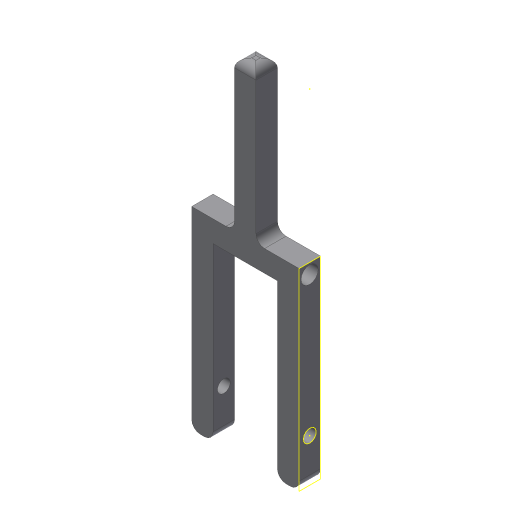
# Autodesk Inventor part: Hebel
Saved by Autodesk Inventor 2023 (Build 270158000, 158)
## iProperties
Created: 2025-01-21
Part Number: Hebel
Material: Generisch
Document SubType Name: Modeling
Designer: abdel
Density: 1 g/cm^3
Appearance: Vorgabe
Author: abdel
Autodesk Inventor part; units mm, degrees
ref_plane "YZ Plane" through (0, 0, 0) normal (1, 0, 0) x (0, 1, 0)
ref_plane "XZ Plane" through (0, 0, 0) normal (0, 1, 0) x (-1, 0, 0)
ref_plane "XY Plane" through (0, 0, 0) normal (0, 0, 1) x (1, 0, 0)
sketch "Skizze1" plane through (0, 0, 0) normal (0, 0, 1) x (1, 0, 0)
  line L0 (-2.5, -2.5) -> (2.5, -2.5)
  line L1 (2.5, -2.5) -> (2.5, 2.5)
  line L2 (2.5, 2.5) -> (-2.5, 2.5)
  line L3 (-2.5, 2.5) -> (-2.5, -2.5)
  line L4 (-2.5, -2.5) -> (2.5, 2.5) construction
  line L5 (2.5, -2.5) -> (-2.5, 2.5) construction
  point P0 (0, 0)
  dimension "d0" = 5
  dimension "d1" = 5
  constraints: 12 end point, 2 midpoint, 2 parallel, 1 horizontal, 1 perpendicular
  measures "d0" distance of L2.end L1.end
  measures "d1" distance of L1.end L0.end
extrude "Extrusion1" add sketch "Skizze1" against normal blind 40
sketch "Skizze3" plane through (-2.5, -2.5, 0) normal (-1, 0, 0) x (0, 0, 1)
  line L0 (0, 5) -> (-40, 5) projected
  line L1 (-40, 0) -> (-40, 5) projected
  line L2 (0, 0) -> (-40, 0) projected
  line L3 (-35, 5) -> (-40, 5)
  line L4 (-40, 5) -> (-40, 0)
  line L5 (-40, 0) -> (-35, 0)
  line L6 (-35, 0) -> (-35, 5)
  line L7 (-35, 5) -> (-40, 0) construction
  line L8 (-40, 5) -> (-35, 0) construction
  point P0 (0, 2.5)
  point P1 (-37.5, 2.5)
  point P2 (-40, 2.5)
  point P3 (-35, 0)
  point P4 (-35, 5)
  dimension "d14" = 5
  dimension "d15" = 5
  constraints: 12 end point, 4 midpoint, 2 parallel, 1 horizontal, 1 perpendicular
  measures "d14" distance of L5.end L4.end
  measures "d15" distance of L4.end L3.end
sketch "Skizze4" plane through (2.5, -2.5, 0) normal (1, 0, 0) x (0, 0, -1)
  line L0 (0, 0) -> (40, 0) projected
  line L1 (40, 5) -> (40, 0) projected
  line L2 (0, 5) -> (40, 5) projected
  line L3 (35, 5) -> (40, 5)
  line L4 (40, 5) -> (40, 0)
  line L5 (40, 0) -> (35, 0)
  line L6 (35, 0) -> (35, 5)
  line L7 (35, 5) -> (40, 0) construction
  line L8 (40, 5) -> (35, 0) construction
  point P0 (0, 2.5)
  point P1 (37.5, 2.5)
  point P2 (40, 2.5)
  point P3 (35, 5)
  point P4 (35, 0)
  dimension "d16" = 5
  dimension "d17" = 5
  constraints: 12 end point, 4 midpoint, 2 parallel, 1 horizontal, 1 perpendicular
  measures "d16" distance of L4.end L5.end
  measures "d17" distance of L3.end L4.end
extrude "Extrusion2" add sketch "Skizze4" along normal blind 10
extrude "Extrusion3" add sketch "Skizze3" along normal blind 10
sketch "Skizze5" plane through (0, 0, -40) normal (0, 0, -1) x (-1, 0, 0)
  line L0 (12.5, -2.5) -> (-12.5, -2.5) projected
  line L1 (12.5, 2.5) -> (12.5, -2.5) projected
  line L2 (-12.5, 2.5) -> (12.5, 2.5) projected
  line L3 (-12.5, -2.5) -> (-12.5, 2.5) projected
  line L4 (12.5, -2.5) -> (7.5, -2.5)
  line L5 (7.5, -2.5) -> (7.5, 2.5)
  line L6 (7.5, 2.5) -> (12.5, 2.5)
  line L7 (12.5, 2.5) -> (12.5, -2.5)
  line L8 (12.5, -2.5) -> (7.5, 2.5) construction
  line L9 (7.5, -2.5) -> (12.5, 2.5) construction
  line L10 (-7.5, 2.5) -> (-12.5, 2.5)
  line L11 (-12.5, 2.5) -> (-12.5, -2.5)
  line L12 (-12.5, -2.5) -> (-7.5, -2.5)
  line L13 (-7.5, -2.5) -> (-7.5, 2.5)
  line L14 (-7.5, 2.5) -> (-12.5, -2.5) construction
  line L15 (-12.5, 2.5) -> (-7.5, -2.5) construction
  point P0 (0, 0)
  point P1 (10, 0)
  point P2 (-10, 0)
  point P3 (12.5, 0)
  point P4 (-12.5, 0)
  point P5 (7.5, 2.5)
  dimension "d22" = 5
  dimension "d23" = 5
  dimension "d24" = 5
  dimension "d25" = 5
  constraints: 24 end point, 8 midpoint, 4 parallel, 2 horizontal, 2 perpendicular
  measures "d22" distance of L5.end L6.end
  measures "d23" distance of L4.end L5.end
  measures "d24" distance of L12.end L11.end
  measures "d25" distance of L11.end L10.end
extrude "Extrusion4" add sketch "Skizze5" along normal blind 40 contours L0 L5 L2 L1 | L0 L3 L2 L13
sketch "Skizze6" plane through (-12.5, -2.5, 0) normal (-1, 0, 0) x (0, 0, 1)
  line L0 (-80, 0) -> (-80, 5) projected
  line L1 (-35, 0) -> (-80, 0) projected
  point P0 (0, 2.5)
  point P1 (-70, 2.5)
  point P2 (-80, 2.5)
  dimension "d35" = 10
  dimension "d36" = 2.5
  constraints: 1 midpoint
  measures "d35" distance of point (-80, 2.5) point (-70, 2.5)
  measures "d36" distance from line of L1 point (-70, 2.5)
hole "Bohrung2" at (-12.5, 0, -70) direction (1, 0, 0) diameter 3 end through all
sketch "Skizze7" plane through (12.5, -2.5, 0) normal (1, 0, 0) x (0, 0, -1)
  circle A0 centre (70, 2.5) radius 1.5 projected
  line L0 (35, 0) -> (80, 0) projected
  line L1 (80, 5) -> (80, 0) projected
  line L2 (35, 5) -> (80, 5) projected
  line L3 (35, 5) -> (35, 0) projected
  point P0 (0, 2.5)
sketch "Skizze8" plane through (-12.5, -2.5, 0) normal (-1, 0, 0) x (0, 0, 1)
  line L0 (-35, 0) -> (-80, 0) projected
  line L1 (-35, 0) -> (-35, 5) projected
  point P0 (0, 2.5)
  point P1 (-37.5, 2.5)
  dimension "d44" = 2.5
  dimension "d45" = 2.5
  measures "d44" distance from line of point (-37.5, 2.5) L1
  measures "d45" distance from line of L0 point (-37.5, 2.5)
hole "Bohrung1" at (-12.5, 0, -37.5) direction (1, 0, 0) diameter 4 end through all
fillet "Rundung1" radius 2 10 edges at (-7.5, 0, -80) (7.5, 0, -80) (-12.5, 0, -80) (12.5, 0, -80) (2.5, 0, 0) (-2.5, 0, 0) (0, 2.5, 0) (0, -2.5, 0) (-2.5, 0, -35) (2.5, 0, -35)
